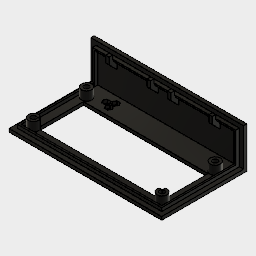
Enclosure Top (Autodesk Fusion 360 design; units mm, degrees)
Autodesk Fusion 360 part; units mm, degrees
sketch "Base" plane through (0, 0, 0) normal (0, 1, 0) x (1, 0, 0)
  line L0 (0, 0) -> (88.9, 0)
  line L1 (88.9, 0) -> (88.9, -49.6)
  line L2 (88.9, -49.6) -> (0, -49.6)
  line L3 (0, -49.6) -> (0, 0)
  line L4 (88.9, 0) -> (0, 0)
  line L5 (0, 0) -> (0, -2)
  line L6 (0, -2) -> (88.9, -2)
  line L7 (88.9, -2) -> (88.9, 0)
  dimension "d1" = 49.6
  dimension "d2" = 88.9
  dimension "d5" = 88.9
  dimension "d6" = 2
  measures "d1" distance of L0.start L2.end
  measures "d2" distance of L0.start L0.end
  measures "d5" distance of L0.end L0.start
  measures "d6" distance of L0.end L6.end
extrude "Extrude1" add sketch "Base" along normal blind 2 contours L1 L2 L3 L6
extrude "Extrude2" add sketch "Base" along normal blind 24 contours L0 L1 L3 L4 L5 L6 L7
sketch "Screen Hole" plane through (0, 2, 0) normal (0, 1, 0) x (-1, 0, 0)
  line L0 (0, 2) -> (0, 49.6)
  line L1 (0, 49.6) -> (-88.9, 49.6)
  line L2 (-88.9, 49.6) -> (-88.9, 2)
  line L3 (-88.9, 2) -> (0, 2)
  line L4 (-80.7, 41.15) -> (-8.2, 41.15)
  line L5 (-8.2, 41.15) -> (-8.2, 14.4)
  line L6 (-8.2, 14.4) -> (-80.7, 14.4)
  line L7 (-80.7, 14.4) -> (-80.7, 41.15)
  line L8 (-80.7, 41.15) -> (-8.2, 14.4) construction
  line L9 (-8.2, 41.15) -> (-80.7, 14.4) construction
  point P0 (-44.45, 27.775)
  point P1 (-44.45, 27.775)
  dimension "d44" = 72.5
  dimension "d45" = 26.75
  measures "d44" distance of L5.end L6.end
  measures "d45" distance of L4.end L5.end
sketch "Face Perimeter" plane through (0, 2, 0) normal (0, 1, 0) x (-1, 0, 0)
  line L0 (0, 2) -> (0, 49.6)
  line L1 (0, 49.6) -> (-88.9, 49.6)
  line L2 (-88.9, 49.6) -> (-88.9, 2)
  line L3 (-88.9, 2) -> (0, 2)
  line L4 (0, 49.6) -> (-2.5, 49.6) construction
  line L5 (-2.5, 49.6) -> (-2.5, 47.1) construction
  line L6 (-2.5, 47.1) -> (0, 47.1) construction
  line L7 (0, 47.1) -> (0, 49.6) construction
  line L8 (-88.9, 49.6) -> (-86.4, 49.6) construction
  line L9 (-86.4, 49.6) -> (-86.4, 47.1) construction
  line L10 (-86.4, 47.1) -> (-88.9, 47.1) construction
  line L11 (-88.9, 47.1) -> (-88.9, 49.6) construction
  line L12 (-88.9, 2) -> (-86.4, 2) construction
  line L13 (0, 2) -> (-2.5, 2) construction
  line L14 (-2.5, 47.1) -> (-3.5, 47.1)
  line L15 (-3.5, 47.1) -> (-3.5, 2)
  line L16 (-3.5, 2) -> (-2.5, 2)
  line L17 (-2.5, 2) -> (-2.5, 47.1)
  line L18 (-86.4, 47.1) -> (-85.4, 47.1)
  line L19 (-85.4, 47.1) -> (-85.4, 2)
  line L20 (-85.4, 2) -> (-86.4, 2)
  line L21 (-86.4, 2) -> (-86.4, 47.1)
  line L22 (-2.5, 47.1) -> (-85.9, 47.1)
  line L23 (-85.9, 47.1) -> (-85.9, 46.1)
  line L24 (-85.9, 46.1) -> (-2.5, 46.1)
  line L25 (-2.5, 46.1) -> (-2.5, 47.1)
  dimension "d17" = 2.5
  dimension "d18" = 2.5
  dimension "d19" = 2.5
  dimension "d20" = 2.5
  dimension "d21" = 2.5
  dimension "d22" = 2.5
  dimension "d23" = 1
  dimension "d24" = 1
  dimension "d25" = 1
  measures "d17" distance of L0.end L6.end
  measures "d18" distance of L0.end L4.end
  measures "d19" distance of L1.end L8.end
  measures "d20" distance of L1.end L10.end
  measures "d21" distance of L2.end L12.end
  measures "d22" distance of L0.start L13.end
  measures "d23" distance of L5.end L14.end
  measures "d24" distance of L9.end L18.end
  measures "d25" distance of L5.end L24.end
extrude "Extrude4" add sketch "Face Perimeter" along normal blind 2 contours L3 L15 L16 L17 L24 | L14 L15 L17 L22 L24 L25 | L3 L18 L19 L20 L21 L23 L24 | L15 L19 L22 L24 | L18 L19 L22 L23 L24
sketch "Screw Holes" plane through (0, 0, 0) normal (0, 1, 0) x (1, 0, 0)
  line L0 (0, -2) -> (6.85, -2) construction
  line L1 (6.85, -2) -> (6.85, -11.3) construction
  line L2 (6.85, -11.3) -> (0, -11.3) construction
  line L3 (0, -11.3) -> (0, -2) construction
  line L4 (88.9, -49.6) -> (81.743, -49.6) construction
  line L5 (81.743, -49.6) -> (81.743, -42.244) construction
  line L6 (81.743, -42.244) -> (88.9, -42.244) construction
  line L7 (88.9, -42.244) -> (88.9, -49.6) construction
  line L8 (6.85, -11.3) -> (81.743, -11.3) construction
  line L9 (81.743, -11.3) -> (81.743, -42.244) construction
  line L10 (81.743, -42.244) -> (6.85, -42.244) construction
  line L11 (6.85, -42.244) -> (6.85, -11.3) construction
  circle A0 centre (6.85, -11.3) radius 1.5
  circle A1 centre (81.743, -11.3) radius 1.5
  circle A2 centre (81.743, -42.244) radius 1.5
  circle A3 centre (6.85, -42.244) radius 1.5
  point P0 (0, -49.6)
  point P1 (88.9, -49.6)
  point P2 (88.9, 0)
  point P3 (0, -2)
  dimension "d36" = 9.3
  dimension "d37" = 6.85
  dimension "d38" = 7.157
  dimension "d39" = 7.356
  dimension "d40" = 3
  dimension "d41" = 3
  dimension "d42" = 3
  dimension "d43" = 3
  measures "d36" distance of P3 L2.end
  measures "d37" distance of P3 L0.end
  measures "d38" distance of P1 L4.end
  measures "d39" distance of P1 L6.end
  measures "d40" diameter of A0
  measures "d41" diameter of A1
  measures "d42" diameter of A2
  measures "d43" diameter of A3
extrude "Extrude5" cut sketch "Screen Hole" against normal blind 2 contours L4 L5 L6 L7
extrude "Extrude6" cut sketch "Screw Holes" along normal blind 2
sketch "Top Perimeter" plane through (0, 0, 2) normal (0, 0, 1) x (1, 0, 0)
  line L0 (85.4, 2) -> (85.4, 4)
  line L1 (85.4, 4) -> (86.4, 4)
  line L2 (86.4, 4) -> (86.4, 2)
  line L3 (86.4, 2) -> (88.9, 2)
  line L4 (88.9, 2) -> (88.9, 24)
  line L5 (88.9, 24) -> (0, 24)
  line L6 (0, 24) -> (0, 2)
  line L7 (0, 2) -> (2.5, 2)
  line L8 (2.5, 2) -> (2.5, 4)
  line L9 (2.5, 4) -> (3.5, 4)
  line L10 (3.5, 4) -> (3.5, 2)
  line L11 (3.5, 2) -> (85.4, 2)
  line L12 (0, 24) -> (3, 24) construction
  line L13 (3, 24) -> (3, 21.5) construction
  line L14 (3, 21.5) -> (0, 21.5) construction
  line L15 (0, 21.5) -> (0, 24) construction
  line L16 (3, 21.5) -> (4, 21.5)
  line L17 (4, 21.5) -> (4, 2)
  line L18 (4, 2) -> (3, 2)
  line L19 (3, 2) -> (3, 21.5)
  line L20 (86.4, 2) -> (85.4, 2)
  line L21 (85.4, 2) -> (85.4, 21.5)
  line L22 (85.4, 21.5) -> (86.4, 21.5)
  line L23 (86.4, 21.5) -> (86.4, 2)
  line L24 (86.4, 21.5) -> (3, 21.5)
  line L25 (3, 21.5) -> (3, 20.5)
  line L26 (3, 20.5) -> (86.4, 20.5)
  line L27 (86.4, 20.5) -> (86.4, 21.5)
  dimension "d50" = 2.5
  dimension "d54" = 1
  dimension "d56" = 1
  dimension "d57" = 1
  measures "d50" distance of L5.end L14.end
  measures "d54" distance of L13.end L16.end
  measures "d56" distance of L2.end L0.start
  measures "d57" distance of L22.end L26.end
extrude "Extrude7" add sketch "Top Perimeter" along normal blind 2 contours L1 L21 L23 L26 | L9 L10 L11 L17 L18 L19 L26 | L17 L21 L24 L26 | L21 L22 L23 L24 L26 L27 | L16 L17 L19 L24 L25 L26
sketch "Decoration" plane through (0, 0, 0) normal (0, 1, 0) x (1, 0, 0)
  line L0 (13, -8) -> (14, -9.7321)
  line L1 (14, -9.7321) -> (16, -9.7321)
  line L2 (16, -9.7321) -> (17, -8)
  line L3 (17, -8) -> (16, -6.2679)
  line L4 (16, -6.2679) -> (14, -6.2679)
  line L5 (14, -6.2679) -> (13, -8)
  line L6 (17.5, -4.2679) -> (16.5, -6)
  line L7 (16.5, -6) -> (17.5, -7.7321)
  line L8 (17.5, -7.7321) -> (19.5, -7.7321)
  line L9 (19.5, -7.7321) -> (20.5, -6)
  line L10 (20.5, -6) -> (19.5, -4.2679)
  line L11 (19.5, -4.2679) -> (17.5, -4.2679)
  line L12 (20.5, -10) -> (19.5, -8.2679)
  line L13 (19.5, -8.2679) -> (17.5, -8.2679)
  line L14 (17.5, -8.2679) -> (16.5, -10)
  line L15 (16.5, -10) -> (17.5, -11.7321)
  line L16 (17.5, -11.7321) -> (19.5, -11.7321)
  line L17 (19.5, -11.7321) -> (20.5, -10)
  point P0 (15, -8)
sketch "Standoff" plane through (0, 2, 0) normal (0, 1, 0) x (-1, 0, 0)
  circle A0 centre (-81.743, 42.244) radius 1.5
  circle A1 centre (-81.743, 11.3) radius 1.5
  circle A2 centre (-6.85, 42.244) radius 1.5
  circle A3 centre (-6.85, 11.3) radius 1.5
  line L0 (-8.2, 41.15) -> (-8.2, 14.4)
  line L1 (-8.2, 14.4) -> (-80.7, 14.4)
  line L2 (-80.7, 14.4) -> (-80.7, 41.15)
  line L3 (-80.7, 41.15) -> (-8.2, 41.15)
  line L4 (-85.4, 46.1) -> (-85.4, 2)
  line L5 (-85.4, 2) -> (-4, 2)
  line L6 (-3.5, 4) -> (-3.5, 46.1)
  line L7 (-3.5, 46.1) -> (-85.4, 46.1)
  circle A4 centre (-6.85, 11.3) radius 3
  circle A5 centre (-81.743, 11.3) radius 3
  circle A6 centre (-6.85, 42.244) radius 3
  circle A7 centre (-81.743, 42.244) radius 3
  line L8 (-4, 4) -> (-3.5, 4)
  line L9 (-4, 2) -> (-4, 4)
  dimension "d62" = 6
  dimension "d63" = 6
  dimension "d64" = 6
  dimension "d65" = 6
  measures "d62" diameter of A4
  measures "d63" diameter of A5
  measures "d64" diameter of A6
  measures "d65" diameter of A7
extrude "Extrude9" add sketch "Standoff" along normal blind 5.25 contours L0 L3 A6 | L2 L3 A7 | A4 | A5 picked at (-8.7748, 40.5363) picked at (-81.0795, 39.8401)
extrude "Extrude10" cut sketch "Decoration" along normal blind 2
delete_face "DeleteFace1" 1 faces at (9.1623, 3.75, 41.15)
extrude "Extrude11" add sketch "Standoff" along normal blind 5.25 contours L0 L3 A6 picked at (-8, 40.5533)
sketch "Screw Pan Depression" plane through (0, 0, 0) normal (0, -1, 0) x (1, 0, 0)
  line L0 (20.5, 6) -> (19.5, 4.2679)
  line L1 (19.5, 4.2679) -> (17.5, 4.2679)
  line L2 (17.5, 4.2679) -> (16.5, 6)
  line L3 (16.5, 6) -> (17.5, 7.7321)
  line L4 (17.5, 7.7321) -> (19.5, 7.7321)
  line L5 (19.5, 7.7321) -> (20.5, 6)
  line L6 (17.5, 11.7321) -> (19.5, 11.7321)
  line L7 (19.5, 11.7321) -> (20.5, 10)
  line L8 (20.5, 10) -> (19.5, 8.2679)
  line L9 (19.5, 8.2679) -> (17.5, 8.2679)
  line L10 (17.5, 8.2679) -> (16.5, 10)
  line L11 (16.5, 10) -> (17.5, 11.7321)
  line L12 (16, 6.2679) -> (14, 6.2679)
  line L13 (14, 6.2679) -> (13, 8)
  line L14 (13, 8) -> (14, 9.7321)
  line L15 (14, 9.7321) -> (16, 9.7321)
  line L16 (16, 9.7321) -> (17, 8)
  line L17 (17, 8) -> (16, 6.2679)
  circle A0 centre (81.743, 42.244) radius 1.5
  circle A1 centre (81.743, 11.3) radius 1.5
  circle A2 centre (6.85, 42.244) radius 1.5
  circle A3 centre (6.85, 11.3) radius 1.5
  line L18 (8.2, 14.4) -> (8.2, 41.15)
  line L19 (8.2, 41.15) -> (80.7, 41.15)
  line L20 (80.7, 41.15) -> (80.7, 14.4)
  line L21 (80.7, 14.4) -> (8.2, 14.4)
  line L22 (0, 49.6) -> (0, 0)
  line L23 (0, 0) -> (88.9, 0)
  line L24 (88.9, 0) -> (88.9, 49.6)
  line L25 (88.9, 49.6) -> (0, 49.6)
  circle A4 centre (6.85, 42.244) radius 2.125
  circle A5 centre (81.743, 42.244) radius 2.125
  circle A6 centre (6.85, 11.3) radius 2.125
  circle A7 centre (81.743, 11.3) radius 2.125
  dimension "d72" = 4.25
  dimension "d73" = 4.25
  dimension "d74" = 4.25
  dimension "d75" = 4.25
  measures "d72" diameter of A4
  measures "d73" diameter of A5
  measures "d74" diameter of A6
  measures "d75" diameter of A7
extrude "Extrude12" cut sketch "Screw Pan Depression" against normal blind 2.25 contours L18 L19 A4 | L19 L20 A5 | A6 | A7 picked at (8.0617, 40.9414) picked at (80.9604, 40.4995)
delete_face "DeleteFace2" 1 faces at (9.8306, 3.75, 42.5846)
delete_face "DeleteFace3" 1 faces at (81.7927, 3.75, 45.2436)
extrude "Extrude13" add sketch "Standoff" along normal blind 5.25 contours L0 L3 A6 | L2 L3 A7 picked at (-8, 40.5533) picked at (-81.0795, 39.8401)
sketch "Latches Uprights" plane through (0, 0, 2) normal (0, 0, 1) x (1, 0, 0)
  line L0 (3, 4) -> (3, 21.5)
  line L1 (3, 21.5) -> (86.4, 21.5)
  line L2 (86.4, 21.5) -> (86.4, 2)
  line L3 (86.4, 2) -> (88.9, 2)
  line L4 (88.9, 2) -> (88.9, 24)
  line L5 (88.9, 24) -> (0, 24)
  line L6 (0, 24) -> (0, 2)
  line L7 (0, 2) -> (2.5, 2)
  line L8 (2.5, 2) -> (2.5, 4)
  line L9 (2.5, 4) -> (3, 4)
  line L10 (14.2474, 21.5) -> (15.2474, 21.5) construction
  line L11 (14.2474, 21.5) -> (13.2474, 21.5) construction
  line L12 (13.2474, 21.5) -> (15.2474, 21.5)
  line L13 (15.2474, 21.5) -> (15.2474, 15.5)
  line L14 (15.2474, 15.5) -> (13.2474, 15.5)
  line L15 (13.2474, 15.5) -> (13.2474, 21.5)
  line L16 (37.2474, 15.5) -> (37.2474, 21.5)
  line L17 (37.2474, 21.5) -> (39.2474, 21.5)
  line L18 (39.2474, 21.5) -> (39.2474, 15.5)
  line L19 (39.2474, 15.5) -> (37.2474, 15.5)
  line L20 (49.2474, 21.5) -> (51.2474, 21.5)
  line L21 (51.2474, 21.5) -> (51.2474, 15.5)
  line L22 (51.2474, 15.5) -> (49.2474, 15.5)
  line L23 (49.2474, 15.5) -> (49.2474, 21.5)
  line L24 (73.2474, 21.5) -> (75.2474, 21.5)
  line L25 (75.2474, 21.5) -> (75.2474, 15.5)
  line L26 (75.2474, 15.5) -> (73.2474, 15.5)
  line L27 (73.2474, 15.5) -> (73.2474, 21.5)
  point P0 (88.9014, 21.5)
  point P1 (0, 21.5)
  point P2 (14.2474, 21.5)
  point P3 (38.2474, 21.5)
  point P4 (50.2474, 21.5)
  point P5 (74.2474, 21.5)
  dimension "d81" = 14.654
  dimension "d82" = 24
  dimension "d83" = 12
  dimension "d84" = 24
  dimension "d85" = 1
  dimension "d86" = 1
  dimension "d87" = 6
  dimension "d88" = 6
  dimension "d89" = 6
  dimension "d90" = 6
  measures "d81" distance of P0 P5
  measures "d82" distance of P4 P5
  measures "d83" distance of P3 P4
  measures "d84" distance of P2 P3
  measures "d85" distance of P2 L10.end
  measures "d86" distance of P2 L11.end
  measures "d87" distance of L11.end L14.end
  measures "d88" distance of L16.end L16.start
  measures "d89" distance of L22.end L20.start
  measures "d90" distance of L24.start L26.end
extrude "Extrude14" cut sketch "Latches Uprights" along normal blind 4.5 contours L1 L12 L13 L14 L15 | L1 L16 L17 L18 L19 | L1 L20 L21 L22 L23 | L1 L24 L25 L26 L27
extrude "Extrude15" add sketch "Latches Uprights" along normal blind 4.5 contours L1 L12 L13 L14 L15 | L1 L16 L17 L18 L19 | L1 L20 L21 L22 L23 | L1 L24 L25 L26 L27
sketch "Latch Fingers" plane through (0, 21.5, 0) normal (0, 1, 0) x (-1, 0, 0)
  line L0 (-86.4, 2) -> (-3, 2)
  line L1 (-3, 2) -> (-3, 4)
  line L2 (-3, 4) -> (-13.2474, 4)
  line L3 (-13.2474, 4) -> (-13.2474, 6.5)
  line L4 (-13.2474, 6.5) -> (-15.2474, 6.5)
  line L5 (-15.2474, 6.5) -> (-15.2474, 4)
  line L6 (-15.2474, 4) -> (-37.2474, 4)
  line L7 (-37.2474, 4) -> (-37.2474, 6.5)
  line L8 (-37.2474, 6.5) -> (-39.2474, 6.5)
  line L9 (-39.2474, 6.5) -> (-39.2474, 4)
  line L10 (-39.2474, 4) -> (-49.2474, 4)
  line L11 (-49.2474, 4) -> (-49.2474, 6.5)
  line L12 (-49.2474, 6.5) -> (-51.2474, 6.5)
  line L13 (-51.2474, 6.5) -> (-51.2474, 4)
  line L14 (-51.2474, 4) -> (-73.2474, 4)
  line L15 (-73.2474, 4) -> (-73.2474, 6.5)
  line L16 (-73.2474, 6.5) -> (-75.2474, 6.5)
  line L17 (-75.2474, 6.5) -> (-75.2474, 4)
  line L18 (-75.2474, 4) -> (-86.4, 4)
  line L19 (-86.4, 4) -> (-86.4, 2)
  line L20 (-75.2474, 6.5) -> (-73.2474, 6.5)
  line L21 (-73.2474, 6.5) -> (-73.2474, 4.5)
  line L22 (-73.2474, 4.5) -> (-75.2474, 4.5)
  line L23 (-75.2474, 4.5) -> (-75.2474, 6.5)
  line L24 (-51.2474, 6.5) -> (-49.2474, 6.5)
  line L25 (-49.2474, 6.5) -> (-49.2474, 4.5)
  line L26 (-49.2474, 4.5) -> (-51.2474, 4.5)
  line L27 (-51.2474, 4.5) -> (-51.2474, 6.5)
  line L28 (-39.2474, 6.5) -> (-37.2474, 6.5)
  line L29 (-37.2474, 6.5) -> (-37.2474, 4.5)
  line L30 (-37.2474, 4.5) -> (-39.2474, 4.5)
  line L31 (-39.2474, 4.5) -> (-39.2474, 6.5)
  line L32 (-15.2474, 6.5) -> (-13.2474, 6.5)
  line L33 (-13.2474, 6.5) -> (-13.2474, 4.5)
  line L34 (-13.2474, 4.5) -> (-15.2474, 4.5)
  line L35 (-15.2474, 4.5) -> (-15.2474, 6.5)
  dimension "d95" = 2
  dimension "d96" = 2
  dimension "d97" = 2
  dimension "d98" = 2
  measures "d95" distance of L16.end L22.end
  measures "d96" distance of L12.end L26.end
  measures "d97" distance of L30.end L8.end
  measures "d98" distance of L34.end L4.end
extrude "Extrude16" add sketch "Latch Fingers" along normal blind 2.5 contours L15 L16 L17 L20 L21 L22 L23 | L3 L4 L5 L32 L33 L34 L35 | L11 L12 L13 L24 L25 L26 L27 | L7 L8 L9 L28 L29 L30 L31
chamfer "Chamfer1" distance 4.5 angle 45 4 edges at (74.2474, 15.5, 6.5) (50.2474, 15.5, 6.5) (38.2474, 15.5, 6.5) (14.2474, 15.5, 6.5)
sketch "Overhang Support" plane through (0, 0, 2) normal (0, 0, 1) x (1, 0, 0)
  line L0 (39.2474, 20.5) -> (39.2474, 15.5)
  line L1 (39.2474, 15.5) -> (37.2474, 15.5)
  line L2 (37.2474, 15.5) -> (37.2474, 20.5)
  line L3 (73.2474, 20.5) -> (51.2474, 20.5)
  line L4 (4, 20.5) -> (4, 2)
  line L5 (4, 2) -> (85.4, 2)
  line L6 (85.4, 2) -> (85.4, 20.5)
  line L7 (75.2474, 20.5) -> (75.2474, 15.5)
  line L8 (75.2474, 15.5) -> (73.2474, 15.5)
  line L9 (73.2474, 15.5) -> (73.2474, 20.5)
  line L10 (51.2474, 20.5) -> (51.2474, 15.5)
  line L11 (51.2474, 15.5) -> (49.2474, 15.5)
  line L12 (49.2474, 15.5) -> (49.2474, 20.5)
  line L13 (15.2474, 20.5) -> (15.2474, 15.5)
  line L14 (15.2474, 15.5) -> (13.2474, 15.5)
  line L15 (13.2474, 15.5) -> (13.2474, 20.5)
  line L16 (73.2474, 20.5) -> (-8.1526, 20.5)
  line L17 (-8.1526, 20.5) -> (-8.1526, 19.5)
  line L18 (-8.1526, 19.5) -> (73.2474, 19.5)
  line L19 (73.2474, 19.5) -> (73.2474, 20.5)
  line L20 (49.2474, 20.5) -> (39.2474, 20.5)
  line L21 (37.2474, 20.5) -> (15.2474, 20.5)
  line L22 (13.2474, 20.5) -> (4, 20.5)
  line L23 (85.4, 20.5) -> (75.2474, 20.5)
  dimension "d118" = 1
  measures "d118" distance of L3.start L18.end
extrude "Extrude20" [rolled back] along distance 1 taper angle 0
